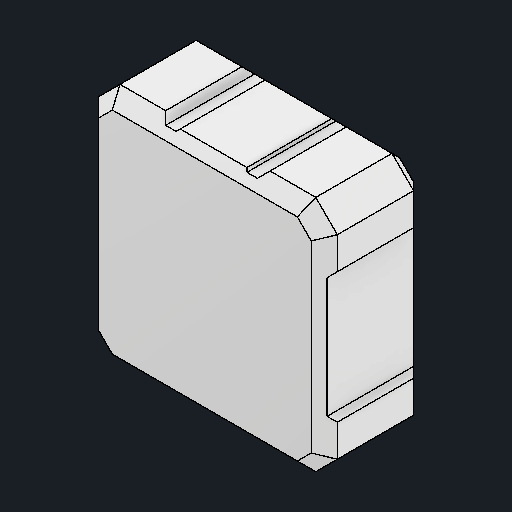
# Autodesk Inventor part: Inclinometer
Saved by Autodesk Inventor 2026.2 (Build 302298000, 298)
## iProperties
Created: 2026-01-19
Part Number: Inclinometer
Material: ABS Plastic
Document SubType Name: Modeling
Designer: JoshuaEah
Density: 1.06 g/cm^3
Appearance: Smooth - White
Author: JoshuaEah
Autodesk Inventor part; units mm, degrees
ref_plane "YZ Plane" through (0, 0, 0) normal (1, 0, 0) x (0, 1, 0)
ref_plane "XZ Plane" through (0, 0, 0) normal (0, 1, 0) x (-1, 0, 0)
ref_plane "XY Plane" through (0, 0, 0) normal (0, 0, 1) x (1, 0, 0)
sketch "Sketch1" plane through (0, 0, 0) normal (0, 0, 1) x (1, 0, 0)
  line L0 (0, 0) -> (58.1152, 0)
  line L1 (58.1152, 0) -> (58.1152, 57.785)
  line L2 (58.1152, 57.785) -> (0, 57.785)
  line L3 (0, 57.785) -> (0, 0)
  line L4 (0, 43.4975) -> (58.1152, 43.4975)
  line L5 (0, 28.8925) -> (58.1152, 28.8925)
  line L6 (0, 14.2875) -> (58.1152, 14.2875)
  line L7 (29.0576, 57.785) -> (29.0576, 0)
  line L8 (16.3576, 57.785) -> (16.3576, 0)
  line L9 (41.7576, 57.785) -> (41.7576, 0)
  line L10 (1.2446, 43.4975) -> (1.2446, 14.2875)
  line L11 (56.8706, 43.4975) -> (56.8706, 14.2875)
  line L12 (16.3576, 56.7436) -> (41.7576, 56.7436)
  line L13 (16.3576, 1.0414) -> (41.7576, 1.0414)
  line L14 (4.9602, 57.785) -> (10.8826, 57.785) construction
  line L15 (0, 52.54) -> (5.245, 57.785)
  line L16 (58.1152, 52.54) -> (52.8702, 57.785)
  line L17 (0, 5.245) -> (5.245, 0)
  line L18 (58.1152, 5.245) -> (52.8702, 0)
  line L19 (41.7576, 56.242) -> (16.3576, 56.242)
  line L20 (41.7576, 1.543) -> (16.3576, 1.543)
  line L21 (41.7576, 57.785) -> (40.2146, 56.242)
  line L22 (16.3576, 57.785) -> (17.9006, 56.242)
  line L23 (41.7576, 0) -> (40.2146, 1.543)
  line L24 (16.3576, 0) -> (17.9006, 1.543)
  line L25 (37.6746, 57.785) -> (37.6746, 56.242)
  line L26 (20.4406, 57.785) -> (20.4406, 56.242)
  line L27 (37.6746, 0) -> (37.6746, 1.543)
  line L28 (20.4406, 0) -> (20.4406, 1.543)
  point P0 (52.8702, 0)
  point P1 (17.399, 1.0414)
  point P2 (40.7162, 1.0414)
  point P3 (17.399, 56.7436)
  point P4 (40.7162, 56.7436)
  point P5 (20.4406, 56.7436)
  point P6 (37.6746, 56.7436)
  point P7 (20.4406, 1.0414)
  point P8 (37.6746, 1.0414)
  dimension "d0" = 58.1152
  dimension "d1" = 57.785
  dimension "d2" = 29.21
  dimension "d3" = 25.4
  dimension "d4" = 55.626
  dimension "d5" = 55.7022
  dimension "d18" = 74.5363
  dimension "d19" = 45
  dimension "d34" = 54.6989
  dimension "d35" = 45
  dimension "d36" = 2.54
  constraints: 58 end point, 25 symmetric about line, 16 point on line, 7 perpendicular, 4 midpoint, 2 horizontal, 2 parallel
  measures "d0" distance of L2.end L1.end
  measures "d1" distance of L1.end L0.end
  measures "d2" diameter of L4 L5
  measures "d3" diameter of L8 L7
  measures "d4" diameter of L10 L7
  measures "d5" diameter of L12 L5
  measures "d18" distance between parallel lines of L18 L15
  measures "d19" angle of L2 L15
  measures "d34" diameter of L19 L5
  measures "d35" angle of L21 L2
  measures "d36" distance from line of L21.end L25
extrude "Extrusion1" add sketch "Sketch1" along normal blind 24.892
extrude "Extrusion2" cut sketch "Sketch1" along normal through all contours L24 L13 L28 L0 | L3 L5 L10 L6 | L28 L13 L7 L0 | L24 L20 L28 L13 | L3 L4 L10 L5 | L7 L13 L27 L0 | L27 L13 L23 L0 | L27 L20 L23 L13 | L2 L26 L12 L22 | L11 L5 L1 L6 | L2 L7 L12 L26 | L12 L26 L19 L22 | L11 L4 L1 L5 | L2 L25 L12 L7 | L25 L12 L21 L19 | L2 L21 L12 L25
extrude "Extrusion3" cut sketch "Sketch1" along normal through all contours L3 L17 L0 | L3 L2 L15 | L18 L1 L0 | L16 L2 L1
chamfer "Chamfer5" distance 3.175 angle 45 8 edges at (2.6225, 55.1625, 24.892) (55.4927, 55.1625, 24.892) (55.4927, 2.6225, 24.892) (2.6225, 2.6225, 24.892) (2.6225, 2.6225, 0) (2.6225, 55.1625, 0) (55.4927, 55.1625, 0) (55.4927, 2.6225, 0)
chamfer "Chamfer6" distance 3.175 angle 45 8 edges at (0, 45.7737, 0) (13.0464, 57.785, 0) (45.0688, 0, 0) (58.1152, 12.0113, 0) (0, 45.7737, 24.892) (13.0464, 57.785, 24.892) (58.1152, 12.0113, 24.892) (45.0688, 0, 24.892)
chamfer "Chamfer7" distance 0.5017 angle 45 4 edges at (37.6746, 56.7436, 12.446) (20.4406, 56.7436, 12.446) (37.6746, 1.0414, 12.446) (20.4406, 1.0414, 12.446)
chamfer "Chamfer8" distance 1.2446 angle 45 4 edges at (58.1152, 43.4975, 12.446) (58.1152, 14.2875, 12.446) (0, 43.4975, 12.446) (0, 14.2875, 12.446)
body "Solid1"
